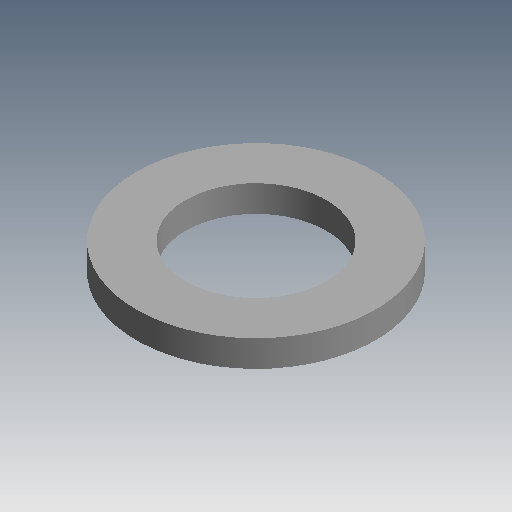
# Autodesk Inventor part: HCBST5w
Saved by Autodesk Inventor 2020 (Build 240168000, 168)
## iProperties
Part Number: HCBST5w
Material: Generic
Catalog Web Link: www.cadenas.de
Description: HCBST_secwasher-Washer Assembled Hexagon Socket Head Cap Screws
Vendor: MISUMI
Document SubType Name: Modeling
Designer: partserver
Manufacturer: MISUMI
Mass: 0.0415554 g
Surface Area: 1.28036 cm^2
Volume: 0.0415554 cm^3
Density: 1 g/cm^3
Appearance: PSOLRGB-192-192-192
Category: PARTsolutions
Company: MISUMI
PSOL_IDENT_0: {$CADENAS_DATA\23d-libs\misumi\metric\38_al_extrusions_blackets\38_accessories\sec_parts\sec_washer.
PSOL_IDENT_1: prj},162 {VTYP=3D},{NB=HCBST5w},{LINA=HCBST5},{NN=HCBST_secwasher},{DATE=30.03.2018 06:53:28},{GEOMD
PSOL_IDENT_2: ATE=13.10.2015 04:19:17},{VERSION=},{LINEID=40},{WBVAR=},{WBNUMERIC=}  {NB=HCBST5w},{LINA=HCBST5},{K
PSOL_IDENT_3: T=DUMMY},{PN=HCBST5},{M=5},{M1=5},{MP=5x0.8},{P=0.800},{D=9},{DD=5.3},{TT=1.0}
NB: HCBST5w
NN: HCBST_secwasher
NT: Washer Assembled Hexagon Socket Head Cap Screws
NBSYN: $PN.w
LINA: HCBST5
CATALOG: Misumi
M: 5
M1: 5
D: 9
DD: 5.3
TT: 1
SUPPLIER: MISUMI
ARTICLENO: HCBST5w
BOMINFO: HCBST5
CREATOR: CADENAS GmbH
Title: HCBST5
Author: Cadenas PARTsolutions
Comments: Washer Assembled Hexagon Socket Head Cap Screws
Autodesk Inventor part; units mm, degrees
sketch "Sketch_2" plane through (0, 0, 0) normal (0, 0, 1) x (1, 0, 0)
  circle A0 centre (0, 0) radius 4.5
  circle A1 centre (0, 0) radius 2.65
  constraints: 2 centre point
extrude "Extrusion1" add sketch "Sketch_2" against normal blind 1
ref_plane "washer_to_bolt_XY" through (0, 0, 0) normal (0, 0, 1) x (1, 0, 0)
ref_plane "washer_to_bolt_YZ" through (0, 0, 0) normal (1, 0, 0) x (0, 1, 0)
ref_plane "washer_to_bolt_ZX" through (0, 0, 0) normal (0, 1, 0) x (0, 0, 1)
body "Solid1"
